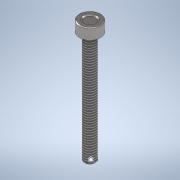
# Autodesk Inventor part: M2
Saved by Autodesk Inventor 2022.2 (Build 262287000, 287)
## iProperties
Created: 2022-08-20
Part Number: M2
Material: Steel, Galvanized
Document SubType Name: Modeling
Designer: ABL
Density: 7.85 g/cm^3
Appearance: Galvanized
Author: ABL
Autodesk Inventor part; units mm, degrees
ref_plane "YZ Plane" through (0, 0, 0) normal (1, 0, 0) x (0, 1, 0)
ref_plane "XZ Plane" through (0, 0, 0) normal (0, 1, 0) x (-1, 0, 0)
ref_plane "XY Plane" through (0, 0, 0) normal (0, 0, 1) x (1, 0, 0)
sketch "Sketch1" plane through (0, 0, 0) normal (0, 0, 1) x (1, 0, 0)
  line L0 (0, 0) -> (0, 22)
  line L1 (0, 22) -> (1.9, 22)
  line L2 (1.9, 22) -> (1.9, 20)
  line L3 (0, 0) -> (1, 0)
  line L4 (1, 0) -> (1, 20)
  line L5 (1, 20) -> (1.9, 20)
  dimension "d0" = 22
  dimension "d1" = 1.9
  dimension "d2" = 2
  dimension "d3" = 1
  dimension "d4" = 20
  constraints: 12 end point, 2 horizontal, 2 vertical, 1 perpendicular
  measures "d0" distance of L0.start L0.end
  measures "d1" distance of L0.end L1.end
  measures "d2" distance of L1.end L2.end
  measures "d3" distance of L0.start L3.end
  measures "d4" distance of L3.end L4.end
revolve "Revolution1" add sketch "Sketch1" angle 360 about axis through (0, 0, 0) along (0, 1, 0)
chamfer "Chamfer1" distance 0.2 angle 45 2 edges at (-1, 0, 0) (-1, 20, 0)
sketch "Sketch2" plane through (0, 22, 0) normal (0, 1, 0) x (1, 0, 0)
  line L0 (1, -0.5774) -> (0, -1.1547)
  line L1 (0, -1.1547) -> (-1, -0.5774)
  line L2 (-1, -0.5774) -> (-1, 0.5774)
  line L3 (-1, 0.5774) -> (0, 1.1547)
  line L4 (0, 1.1547) -> (1, 0.5774)
  line L5 (1, 0.5774) -> (1, -0.5774)
  line L6 (-1, -0.5774) -> (1, 0.5774) construction
  point P0 (0, 0)
  point P1 (0, 0)
  dimension "d8" = 2
  dimension "d24" = 2.3094
  constraints: 14 end point, 1 coincident, 1 vertical, 13 other
  measures "d8" distance between parallel lines of L5 L2
  measures "d24" distance of L1.end L4.end
extrude "HexagonSocket" [suppressed]
ref_plane "Work Plane3" through (0, 20.8, 0) normal (0, 1, 0) x (1, 0, 0)
sketch "Sketch10" plane through (0, 20.8, 0) normal (0, 1, 0) x (1, 0, 0)
  circle A0 centre (0, 0) radius 0.1875
  dimension "d70" = 0.375
  constraints: 1 centre point, 1 coincident
  measures "d70" diameter of A0
feature "Socket_bottomTaper" [suppressed]
sketch "Sketch4" plane through (0, 22, 0) normal (0, 1, 0) x (1, 0, 0)
  circle A0 centre (0, 0) radius 1.2047
  dimension "d25" = 2.4094
  constraints: 1 centre point, 1 coincident
  measures "d25" diameter of A0
ref_plane "Work Plane1" through (0, 21.8, 0) normal (0, 1, 0) x (1, 0, 0)
sketch "Sketch5" plane through (0, 21.8, 0) normal (0, 1, 0) x (1, 0, 0)
  circle A0 centre (0, 0) radius 1
  dimension "d27" = 2
  constraints: 1 centre point, 1 coincident
  measures "d27" diameter of A0
ref_plane "Work Plane2" through (0, 22, 0) normal (0, 1, 0) x (1, 0, 0)
loft "Socket_topTaper" cut profiles "Sketch4", "Sketch5"
chamfer "Chamfer3" distance 0.1 angle 60 2 edges at (-1.9, 22, 0) (-1.9, 20, 0) measured on face at (-1.9, 20.5, 0) measured on face at (-1.9, 21.5, 0)
sketch "Sketch6" plane through (0, 21.8, 0) normal (0, 1, 0) x (1, 0, 0)
  line L0 (0, 0) -> (-1.9, 0) construction
  line L1 (0, 0) -> (-2, 0) construction
  line L2 (-2, 0) -> (-2, 0.2)
  line L3 (-2, 0) -> (-2, -0.2)
  line L4 (-2, -0.2) -> (-1.8894, -0.2)
  line L5 (-2, 0.2) -> (-1.8894, 0.2)
  line L6 (-1.8894, -0.2) -> (-1.8894, 0.2)
  circle A0 centre (0, 0) radius 1.9 construction
  dimension "d34" = 1.9
  dimension "d35" = 2
  dimension "d36" = 0.2
  dimension "d37" = 0.2
  dimension "d40" = 0.1106
  dimension "d75" = 3.8
  constraints: 14 end point, 3 horizontal, 2 point on circle, 2 vertical, 1 centre point, 1 coincident, 1 perpendicular
  measures "d34" distance of L0.start L0.end
  measures "d35" distance of L0.start L1.end
  measures "d36" distance of L1.end L2.end
  measures "d37" distance of L1.end L3.end
  measures "d40" distance of L2.end L5.end
  measures "d75" diameter of A0
extrude "Grip Knurling" [suppressed]
fillet "Fillet3" [suppressed]
pattern_circular "Circular Pattern1" [suppressed]
pattern_circular "Circular Pattern2" [suppressed]
sketch "Sketch7" plane through (0, 0, 0) normal (0, 0, 1) x (1, 0, 0)
  line L0 (-1, 0.2) -> (1, 0.2) construction
  line L1 (-1, -0.2571) -> (-0.7393, -0.4077)
  line L2 (-0.7393, -0.5066) -> (-1, -0.6571)
  line L3 (-1, -0.6571) -> (-1, -0.2571)
  arc A0 (-0.7393, -0.5066) -> (-0.7393, -0.4077) centre (-0.7679, -0.4571) ccw
  point P0 (0, 0)
  point P1 (-0.8845, -0.4571)
  point P2 (-0.6536, -0.4571)
  dimension "d53" = 0.4
  dimension "d54" = 0.4571
  dimension "d55" = 0
  dimension "d56" = 0.0571
  constraints: 6 end point, 2 point on circle, 2 point on line, 2 tangent, 1 centre point, 1 coincident, 1 vertical, 7 other
  measures "d53" distance of L2.end L1.start
  measures "d54" distance from line of L0 L1.start
  measures "d55" distance from line of point (-1, 0.2) L3
  measures "d56" radius of A0
coil "Coil1" [suppressed]
thread "Thread1" size "M2x0.4" class "6g" standard "ISO Metric profile" full length
sketch "Sketch8" plane through (0.7071, 19.3429, 0.7071) normal (-0.7071068, 0, 0.7071068) x (0.7071068, 0, 0.7071068)
  line L0 (0, 0.4) -> (0, 0) projected
  line L1 (-1, -23.932) -> (-1, 7.0887) projected
  point P0 (-1, -19.3429)
  constraints: 1 vertical alignment, 2 other
revolve "Revolution2" [suppressed]
equation "\"d1\" = 0.5 * headDiameter"
equation "\"d2\" = headHeight"
equation "\"d3\" = 0.5 * shaftDiameter"
equation "\"d21\" = d12"
equation "\"d8\" = shaftDiameter"
equation "\"d27\" = shaftDiameter"
equation "\"shaftDiameter\" = 2"
equation "\"headHeight\" = 2"
equation "\"headDiameter\" = 3.8"
equation "\"gap\" = 0.1"
equation "\"airgap\" = 0.4"
equation "\"wallgap\" = 2"
equation "\"printingLayerHeight\" = 0.2"
equation "\"driveMagnet_height\" = 5"
equation "\"halbachMagnet_height\" = 3"
equation "\"rotorBandBolt_diameter\" = 2"
equation "\"rotorBandBolt_headDiameter\" = 3.98"
equation "\"rotorBandBolt_headHeight\" = 2"
equation "\"rotorBandHexNut_sideToSide\" = 4"
equation "\"rotorBandHexNut_height\" = 1.2"
equation "\"rotorBandSquareNut_sideLength\" = 4"
equation "\"rotorBandSquareNut_height\" = 1.2"
equation "\"sensorMagnet_diameter\" = 5"
equation "\"sensorMagnet_height\" = 2.66667"
equation "\"sensorMagnet_ringRadius\" = 0.5 * driveMagnet_centerSpacingRadius + 2 * wallgap"
equation "\"rotorRadius\" = 2 * gap + driveMagnet_centerSpacingRadius + driveMagnet_length + wallgap"
equation "\"rotor_mountingLipHeight\" = 0.5 * statorThickness"
equation "\"flangeBearing_innerDiameter\" = shaftDiameter"
equation "\"flangeBearing_outerDiameter\" = 16"
equation "\"flangeBearing_flangeDiameter\" = 18"
equation "\"flangeBearing_height\" = 5"
equation "\"flangeBearing_flangeHeight\" = 1"
equation "\"magnetWire_outerDiameter\" = 0.8128"
equation "\"coilThickness\" = 12"
equation "\"statorThickness\" = coilThickness + 2 * wallgap"
equation "\"rotorBandThickness\" = wallgap + rotorBandBolt_headHeight + gap"
equation "\"flangeCoupling_innerDiameter\" = shaftDiameter"
equation "\"flangeCoupling_collarOuterDiameter\" = 16"
equation "\"flangeCoupling_flangeDiameter\" = 32"
equation "\"flangeCoupling_flangeHeight\" = 3.1"
equation "\"flangeCoupling_height\" = flangeCoupling_collarHeight + flangeCoupling_flangeHeight"
equation "\"flangeCoupling_mountHoleDiameter\" = 3.9"
equation "\"flangeCoupling_mountHoleEdgeToEdge\" = 2.05"
equation "\"statorRadius\" = driveMagnet_length + driveMagnet_centerSpacingRadius + 2 * gap"
equation "\"statorMountBolt_diameter\" = 4"
equation "\"statorMountBolt_headDiameter\" = 7"
equation "\"statorMountBolt_headHeight\" = 4"
equation "\"statorMountBolt_shaftLength\" = coilThickness + flangeCoupling_flangeHeight + wallgap"
equation "\"statorMountHexNut_sideToSide\" = 8"
equation "\"statorMountHexNut_height\" = 4"
equation "\"coil_percentCoverage\" = 0.6"
equation "\"statorSpokeDegrees\" = 4deg"
equation "\"statorCoilBolt_diameter\" = 2"
equation "\"statorCoilBolt_headDiameter\" = 3.98"
equation "\"statorCoilBolt_headHeight\" = 2"
equation "\"statorCoilBolt_shaftLength\" = coilThickness"
equation "\"statorCoilHexNut_sideToSide\" = 4"
equation "\"statorCoilHexNut_height\" = 1.2"
equation "\"circuitBoard_height\" = 1.6"
equation "\"hallEffectSensor_height\" = 1.1"
equation "\"hallEffectSensor_length\" = 3"
equation "\"hallEffectSensor_width\" = 1.6"
equation "\"hallEffectSensor_pinLength\" = 0.6"
equation "\"circuitboardMountBolt_diameter\" = 2"
equation "\"circuitboardMountBolt_headDiameter\" = 3.98"
equation "\"circuitboardMountBolt_headHeight\" = 2"
equation "\"circuitboardMountBolt_shaftLength\" = coilThickness"
equation "\"circuitboardMountHexNut_sideToSide\" = 4"
equation "\"circuitboardMountHexNut_height\" = 1.2"
equation "\"statorShellBolt_diameter\" = 3"
equation "\"statorShellBolt_headDiameter\" = 5.68"
equation "\"statorShellBolt_headHeight\" = 3"
equation "\"statorShellBolt_shaftLength\" = statorThickness - statorShellBolt_countersinkDepth"
equation "\"statorShellHexNut_sideToSide\" = 5.3"
equation "\"statorShellHexNut_height\" = 2.3"
equation "\"d26\" = -d12"
equation "\"threadDesignation\" = 0.4"
equation "\"socketSize\" = 1.5"
equation "\"chamferSize\" = 0.2"
equation "\"keyEngagementDepth\" = 1"
equation "\"d12\" = 0.2"
equation "\"driveMagnet_centerSpacingRadius\" = 38.96113"
equation "\"driveMagnet_length\" = 60"
equation "\"flangeCoupling_collarHeight\" = 10"
equation "\"statorShellBolt_countersinkDepth\" = 3.4"
